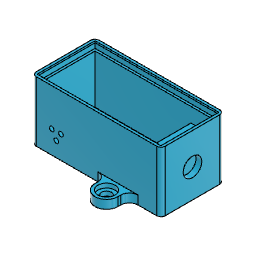
connecteur_ILS_KOSMOS3-0 (Autodesk Fusion 360 design; units mm, degrees)
Autodesk Fusion 360 part; units mm, degrees
sketch "Esquisse1" plane through (0, 0, 0) normal (0, 0, 1) x (1, 0, 0)
  line L0 (0, 0) -> (45, 0)
  line L1 (45, 0) -> (45, 22)
  line L2 (45, 22) -> (0, 22)
  line L3 (0, 22) -> (0, 0)
  dimension "d1" = 22
  dimension "d2" = 45
  constraint horizontal L0
  constraint vertical L1
  constraint horizontal L2
  constraint vertical L3
  constraint coincident L0.start L3.end
  measures "d1" distance of L0.start L2.end
  measures "d2" distance of L0.start L0.end
extrude "Extrusion1" add sketch "Esquisse1" along normal blind 2
sketch "Esquisse2" plane through (0, 0, 2) normal (0, 0, 1) x (-1, 0, 0)
  line L0 (0, 0) -> (-45, 0)
  line L1 (-45, -22) -> (0, -22)
  line L2 (0, -22) -> (0, 0)
  line L3 (0, 0) -> (-45, 0)
  line L4 (-45, 0) -> (-45, -22)
  line L5 (-45, -22) -> (0, -22)
  line L6 (0, -22) -> (0, 0)
  line L7 (-2, -2) -> (-43, -2)
  line L8 (-43, -2) -> (-43, -20)
  line L9 (-43, -20) -> (-2, -20)
  line L10 (-2, -20) -> (-2, -2)
  dimension "d62" = -2
  constraint horizontal L3
  constraint vertical L4
  constraint horizontal L5
  constraint vertical L6
  constraint coincident L1.start L4.end
  constraint coincident L0.start L2.end
extrude "Extrusion2" add sketch "Esquisse2" along normal blind 19
sketch "Esquisse3" plane through (0, 0, 0) normal (0, -1, 0) x (1, 0, 0)
  line L0 (-22, 0) -> (0, 0)
  line L1 (0, 0) -> (0, 21)
  line L2 (0, 21) -> (-22, 21)
  line L3 (17, 7) -> (0, 7) construction
  circle A0 centre (8.5, 7) radius 1.85 construction
  circle A1 centre (8.5014, 5.15) radius 0.8
  circle A2 centre (10.1014, 7.9263) radius 0.8
  circle A3 centre (6.8971, 7.9237) radius 0.8
  line L4 (-22, 21) -> (-22, 0)
  line L5 (0, 0) -> (45, 0)
  line L6 (45, 0) -> (45, 21)
  line L7 (45, 21) -> (0, 21)
  line L8 (0, 21) -> (0, 0)
  dimension "d11" = 7
  dimension "d12" = 3.7
  dimension "d13" = 1.6
  dimension "d15" = 360
  constraint coincident L1 L3.end
  constraint perpendicular L1 L3
  constraint midpoint L3 A0.centre
  constraint coincident A0 A1.centre
  measures "d11" distance of L0 L3
  measures "d12" diameter of A0
  measures "d13" diameter of A1
extrude "Extrusion3" cut sketch "Esquisse3" against normal blind 2 contours A1 | A2 | A3
sketch "Esquisse5" plane through (45, 0, 0) normal (1, 0, 0) x (0, 1, 0)
  line L0 (0, 0) -> (22, 0)
  line L1 (22, 0) -> (22, 21)
  line L2 (22, 21) -> (0, 21)
  line L3 (0, 21) -> (0, 0)
  circle A0 centre (11, 10) radius 3.25
  circle A1 centre (11, 10) radius 2
  dimension "d24" = 6.5
  dimension "d28" = 11
  dimension "d29" = 10
  dimension "d36" = 4
  constraint concentric A0 A1
  measures "d24" diameter of A0
  measures "d28" distance of L3 A0.centre
  measures "d29" distance of L0 A0.centre
  measures "d36" diameter of A1
sketch "Esquisse6" plane through (0, 0, 2) normal (0, 0, 1) x (-1, 0, 0)
  line L0 (-45, -20) -> (-35, -20)
  line L1 (-35, -20) -> (-35, -2)
  line L2 (-35, -2) -> (-45, -2)
  line L3 (-45, -2) -> (-45, -20)
  line L4 (-2, -2) -> (-43, -2)
  line L5 (-43, -2) -> (-43, -20)
  line L6 (-43, -20) -> (-2, -20)
  line L7 (-2, -20) -> (-2, -2)
  dimension "d25" = 10
  constraint horizontal L0
  constraint vertical L1
  constraint horizontal L2
  constraint vertical L3
  measures "d25" distance of L0.start L0.end
extrude "Extrusion5" add sketch "Esquisse6" along normal blind 12 contours L0 L2 L3 L5 | L0 L1 L2 L4 L5 L6
extrude "Extrusion6" cut sketch "Esquisse5" against normal blind 11.5 contours A0 | A1
sketch "Esquisse7" plane through (0, 0, 14) normal (0, 0, 1) x (-1, 0, 0)
  line L0 (-35, -20) -> (-35, -2)
  line L1 (-45, -20) -> (-45, -2)
  line L2 (-45, -20) -> (-39, -20)
  line L3 (-39, -20) -> (-39, -2)
  line L4 (-39, -2) -> (-45, -2)
  line L5 (-45, -2) -> (-45, -20)
  line L6 (-43, -2) -> (-43, -20)
  line L7 (-43, -20) -> (-35, -20)
  line L8 (-35, -2) -> (-43, -2)
  dimension "d35" = 6
  constraint vertical L1
  constraint horizontal L2
  constraint vertical L3
  constraint horizontal L4
  constraint vertical L5
  measures "d35" distance of L1.start L2.end
extrude "Extrusion7" cut sketch "Esquisse7" against normal blind 13 contours L2 L3 L4 L6 L7 L8
sketch "Esquisse8" plane through (39, 0, 0) normal (1, 0, 0) x (0, 1, 0)
  line L0 (20, 14) -> (2, 14)
  line L1 (2, 14) -> (2, 1)
  line L2 (2, 1) -> (20, 1)
  line L3 (20, 1) -> (20, 14)
  circle A0 centre (11, 10) radius 3.25
sketch "Esquisse9" plane through (0, 0, 0) normal (0, 0, -1) x (1, 0, 0)
  line L0 (45, 0) -> (0, 0)
  line L1 (0, 0) -> (0, -22)
  line L2 (0, -22) -> (45, -22)
  line L3 (45, -22) -> (45, 0)
  line L4 (26, 0) -> (34, 0)
  line L5 (34, 0) -> (34, 8)
  line L6 (34, 8) -> (26, 8)
  line L7 (26, 8) -> (26, 0)
  line L8 (30, 0) -> (30, 8) construction
  line L9 (45, -11) -> (5, -11) construction
  line L10 (34, -22) -> (34, -30)
  line L11 (34, -30) -> (26, -30)
  line L12 (26, -30) -> (26, -22)
  line L13 (26, -22) -> (34, -22)
  circle A0 centre (30, 4) radius 1.7
  circle A1 centre (30, -26) radius 1.7
  dimension "d39" = 8
  dimension "d40" = 8
  dimension "d41" = 15
  dimension "d44" = 3.4
  constraint horizontal L4
  constraint vertical L5
  constraint horizontal L6
  constraint vertical L7
  constraint coincident L0 L4.start
  constraint midpoint L4 L8.start
  constraint midpoint L6 L8.end
  constraint midpoint L3 L9.start
  constraint perpendicular L1 L9
  constraint symmetric L4.start L9 L12.end
  constraint symmetric L4.end L9 L10.start
  constraint symmetric L5.end L9 L10.end
  constraint symmetric L6.end L9 L11.end
  constraint midpoint L8 A0.centre
  constraint symmetric L9 A0 A1
  measures "d39" distance of L4.start L4.end
  measures "d40" distance of L4.start L6.end
  measures "d41" distance of L3 L8
  measures "d44" diameter of A0
extrude "Extrusion9" add sketch "Esquisse9" against normal blind 3 contours L0 L4 L5 L6 L7 | L2 L10 L11 L12 L13
fillet "Congé1" radius 4 4 edges at (34, -8, 1.5) (26, -8, 1.5) (34, 30, 1.5) (26, 30, 1.5)
fillet "Congé2" radius 3 4 edges at (34, 0, 1.5) (34, 22, 1.5) (26, 22, 1.5) (26, 0, 1.5)
sketch "Esquisse10" plane through (0, 0, 21) normal (0, 0, 1) x (-1, 0, 0)
  line L0 (-2, -20) -> (-43, -20)
  line L1 (-43, -2) -> (-2, -2)
  line L2 (0, -22) -> (0, 0)
  line L3 (0, 0) -> (-45, 0)
  line L4 (-45, 0) -> (-45, -22)
  line L5 (-45, -22) -> (0, -22)
  line L6 (-2, -2) -> (-2, -20)
  line L7 (-43, -20) -> (-43, -2)
  line L8 (-1.2, -20.8) -> (-43.8, -20.8)
  line L9 (-43.8, -20.8) -> (-43.8, -1.2)
  line L10 (-43.8, -1.2) -> (-1.2, -1.2)
  line L11 (-1.2, -1.2) -> (-1.2, -20.8)
  dimension "d63" = -0.8
extrude "Extrusion10" cut sketch "Esquisse10" against normal blind 2 contours L8 L9 L10 L11
chamfer "Chanfrein1" distance 0.3 angle 45 4 edges at (22.5, 20.8, 21) (1.2, 11, 21) (22.5, 1.2, 21) (43.8, 11, 21)
fillet "Congé3" radius 1.5 4 edges at (0, 0, 10.5) (0, 22, 10.5) (45, 0, 10.5) (45, 22, 10.5)
chamfer "Chanfrein2" distance 0.5 angle 45 2 edges at (39, 11, 14) (35, 11, 14)
hole "Perçage1" at (30, -4, 3) direction (0, 0, -1) diameter 6 depth 1.5 tip angle 180
hole "Perçage2" at (30, 26, 3) direction (0, 0, -1) diameter 6 depth 1.5 tip angle 180
